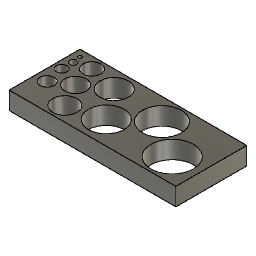
3d hole test v1 (Autodesk Fusion 360 design; units mm, degrees)
Autodesk Fusion 360 part; units mm, degrees
sketch "Sketch1" plane through (0, 0, 0) normal (0, 0, 1) x (1, 0, 0)
  line L0 (0, 0) -> (100, 0)
  line L1 (100, 0) -> (100, 20)
  line L2 (100, 20) -> (0, 20)
  line L3 (0, 20) -> (0, 0)
  dimension "d1" = 100
  dimension "d2" = 20
  constraint horizontal L0
  constraint vertical L1
  constraint horizontal L2
  constraint vertical L3
  constraint coincident L0.start L3.end
  measures "d1" distance of L0.start L0.end
  measures "d2" distance of L0.start L2.end
extrude "Extrude1" add sketch "Sketch1" along normal blind 5
hole "Hole1" at (1.8854, 18.11, 5) direction (0, 0, -1) diameter 1 depth 14.8 tip angle 118
hole "Hole2" at (2.2487, 15.7828, 5) direction (0, 0, -1) diameter 2 depth 14.8 tip angle 118
hole "Hole3" at (2.1769, 12.6179, 5) direction (0, 0, -1) diameter 3 depth 14.8 tip angle 118
hole "Hole4" at (3.2238, 7.4785, 5) direction (0, 0, -1) diameter 4 depth 14.8 tip angle 118
hole "Hole5" at (6.5051, 16.8379, 5) direction (0, 0, -1) diameter 5 depth 14.8 tip angle 118
hole "Hole6" at (8.1033, 10.6225, 5) direction (0, 0, -1) diameter 6 depth 14.8 tip angle 118
hole "Hole7" at (11.6005, 4.1001, 5) direction (0, 0, -1) diameter 6.8 depth 14.8 tip angle 118
hole "Hole8" at (14.5542, 15.0512, 5) direction (0, 0, -1) diameter 8 depth 14.8 tip angle 118
hole "Hole9" at (20.8311, 6.5383, 5) direction (0, 0, -1) diameter 10 depth 14.8 tip angle 118
hole "Hole10" at (29.2038, 13.866, 5) direction (0, 0, -1) diameter 11 depth 14.8 tip angle 118
hole "Hole11" at (39.2107, 6.7415, 5) direction (0, 0, -1) diameter 12 depth 14.8 tip angle 118
move_face "OffsetFaces1" offset -53 1 faces at (100, 6.6667, 1.6667)
thread "Thread12" [rolled back]
thread "Thread1" [rolled back]
thread "Thread2" [rolled back]
thread "Thread3" [rolled back]
thread "Thread4" [rolled back]
thread "Thread5" [rolled back]
thread "Thread6" [rolled back]
thread "Thread7" [rolled back]
thread "Thread8" [rolled back]
thread "Thread9" [rolled back]
thread "Thread10" [rolled back]
thread "Thread11" [rolled back]
